# Autodesk Inventor part: Zahnriemen
Saved by Autodesk Inventor 2016 (Build 200138000, 138)
## iProperties
Created: 2015-08-24
Part Number: Zahnriemen
Material: Rubber
Document SubType Name: Modeling
Designer: 4ndreas
Density: 1 g/cm^3
Appearance: Rubber - Black - Version 1.1
CustomPartVersion: 1
Author: 4ndreas
Autodesk Inventor part; units mm, degrees
sketch "Skizzenpfad" plane through (0, 0, 0) normal (0, 0, 1) x (1, 0, 0)
  arc A0 (-167.1568, 34.6562) -> (-166.9425, -34.4518) centre (-200, 0) ccw
  arc A1 (-136.8151, 5.9017) -> (-131.5827, 3.995) centre (-132, 10.9825) ccw
  arc A2 (-101.5827, 5.7868) -> (-98.3744, 6.7864) centre (-102, 12.7743) ccw
  arc A3 (-93.0707, -9.8477) -> (-91.5947, 10.8915) centre (-85, 0) ccw
  arc A4 (-97.5629, -6.1661) -> (-101.7772, -4.5838) centre (-102, -11.5802) ccw
  arc A5 (-131.7772, -3.6283) -> (-136.8465, -5.5739) centre (-132, -10.6248) ccw
  line L0 (-136.8465, -5.5739) -> (-166.9425, -34.4518)
  line L1 (-167.1568, 34.6562) -> (-136.8151, 5.9017)
  line L2 (-131.5827, 3.995) -> (-101.5827, 5.7868)
  line L3 (-98.3744, 6.7864) -> (-91.5947, 10.8915)
  line L4 (-93.0707, -9.8477) -> (-97.5629, -6.1661)
  line L5 (-101.7772, -4.5838) -> (-131.7772, -3.6283)
  constraints: 12 end point, 12 point on circle, 6 centre point
ref_plane "Querschnittsebene" through (-166.9425, -34.4518, 0) normal (0.7216, 0.6924, 0) x (0, 0, 1)
ref_plane "Arbeitsebene2" through (-200, 0, 0) normal (-1, 0, 0) x (0, 0, 1)
ref_plane "Arbeitsebene3" through (-85, 0, 0) normal (-0.987, -0.1605, 0) x (0, 0, 1)
sketch "Querschnitt" plane through (-166.9425, -34.4518, 0) normal (0.7216, 0.6924, 0) x (0, 0, 1)
  line L0 (-5, 0.5) -> (5, 0.5)
  line L1 (5, 0.5) -> (5, -0.5)
  line L2 (5, -0.5) -> (-5, -0.5)
  line L3 (-5, -0.5) -> (-5, 0.5)
  line L4 (-5, 0) -> (5, 0) construction
  point P0 (0, 0)
  point P1 (0, 0)
  dimension "d0" = 10
  dimension "d4" = 0.5
  dimension "d5" = 0.5
  constraints: 10 end point, 3 midpoint, 2 parallel, 1 coincident, 1 horizontal, 1 perpendicular, 1 other
  measures "d0" distance between parallel lines of L1 L3
  measures "d4" distance between parallel lines of L2 L4
  measures "d5" distance between parallel lines of L4 L0
sweep "Riemen" add profiles "Querschnitt" path "Skizzenpfad"
equation "\"d0\" = da_B"
equation "\"d4\" = da_a"
equation "\"d5\" = da_a2"
equation "\"da_B\" = 10"
equation "\"da_pb\" = 5"
equation "\"da_L\" = 455"
equation "\"da_a\" = 0.5"
equation "\"da_S\" = 2.65"
equation "\"da_Beta\" = 20deg"
equation "\"da_Ht\" = 1.2"
equation "\"da_H\" = 2.2"
equation "\"da_a2\" = 0.5"
body "Solid1"
